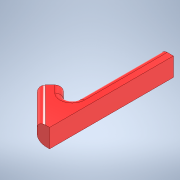
# Autodesk Inventor part: AntennaAdapter
Saved by Autodesk Inventor 2022 (Build 260153000, 153)
## iProperties
Created: 2022-04-08
Part Number: AntennaAdapter
Material: ABS Plastic
Document SubType Name: Modeling
Designer: Sergei
Density: 1.06 g/cm^3
Appearance: Light Red
Author: Sergei
Autodesk Inventor part; units mm, degrees
ref_plane "YZ Plane" through (0, 0, 0) normal (1, 0, 0) x (0, 1, 0)
ref_plane "XZ Plane" through (0, 0, 0) normal (0, 1, 0) x (-1, 0, 0)
ref_plane "XY Plane" through (0, 0, 0) normal (0, 0, 1) x (1, 0, 0)
sketch "Sketch1" plane through (0, 0, 0) normal (0, 1, 0) x (-1, 0, 0)
  line L0 (0, 0) -> (0, -40)
  line L1 (0, -40) -> (4, -40)
  line L2 (4, -40) -> (4, -8.4853)
  line L3 (4, -8.4853) -> (9.6569, -14.1421)
  line L4 (9.6569, -14.1421) -> (13.8995, -9.8995)
  line L5 (13.8995, -9.8995) -> (4, 0)
  line L6 (4, 0) -> (0, 0)
  dimension "d0" = 45
  dimension "d1" = 4
  dimension "d2" = 40
  dimension "d12" = 6
  dimension "d13" = 8
  dimension "d14" = 4
  constraints: 14 end point, 3 perpendicular, 1 horizontal, 1 parallel, 1 vertical
  measures "d0" angle of L2 L3
  measures "d1" distance of L0.end L1.end
  measures "d2" distance of L0.start L0.end
  measures "d12" distance of L3.end L4.end
  measures "d13" distance of L2.end L3.end
  measures "d14" distance of L5.end L0.start
extrude "Extrusion1" add sketch "Sketch1" along normal blind 6
sketch "Sketch2" plane through (-13.8995, 0, -9.8995) normal (-0.7071, 0, -0.7071) x (-0.7071, 0, 0.7071)
  line L0 (-2.8284, 0) -> (-2.8284, 6) projected
  line L1 (-6, 0) -> (0, 0) projected
  line L2 (0, 0) -> (0, 6) projected
  line L3 (-6, 6) -> (0, 6) projected
  line L4 (-6, 0) -> (-6, 6) projected
  circle A0 centre (-3.416, 3) radius 0.65
  dimension "d5" = 1.3
  dimension "d6" = 3
  constraints: 1 centre point
  measures "d5" diameter of A0
  measures "d6" distance from line of L1 A0.centre
extrude "Extrusion2" cut sketch "Sketch2" against normal blind 15 contours A0 L0 | L0 A0
fillet "Fillet1" radius 2 1 edges at (-4, 3, -8.4853)
fillet "Fillet2" radius 2 6 edges at (-8.5355, 6, -13.0208) (-4, 6, -26.6569) (-8.5355, 0, -13.0208) (-4, 0, -26.6569) (-8.9497, 6, -4.9497) (-8.9497, 0, -4.9497)
body "Solid1"
